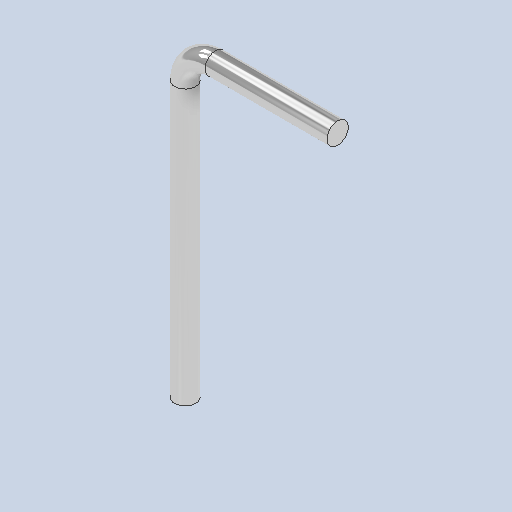
# Autodesk Inventor part: TorsOsc-202511-pin
Saved by Autodesk Inventor 2026 (Build 300175050, 175E)
## iProperties
Created: 2025-12-01
Part Number: TorsOsc-202511-pin
Material: Nickel-Copper Alloy 400
Document SubType Name: Modeling
Designer: schanen
Density: 8.83 g/cm^3
Appearance: Chrome - Polished
Author: schanen
Autodesk Inventor part; units mm, degrees
ref_plane "YZ Plane" through (0, 0, 0) normal (1, 0, 0) x (0, 1, 0)
ref_plane "XZ Plane" through (0, 0, 0) normal (0, 1, 0) x (-1, 0, 0)
ref_plane "XY Plane" through (0, 0, 0) normal (0, 0, 1) x (1, 0, 0)
sketch "Sketch1" plane through (0, 0, 0) normal (0, 0, 1) x (1, 0, 0)
  line L0 (0, 0) -> (0, 9)
  line L1 (1, 10) -> (5, 10)
  arc A0 (1, 10) -> (0, 9) centre (1, 9) ccw
  point P0 (0, 10)
  dimension "d0" = 5
  dimension "d1" = 10
  dimension "d2" = 1
  constraints: 4 end point, 2 point on circle, 2 point on line, 2 tangent, 1 centre point, 1 perpendicular, 1 vertical
  measures "d0" distance of point (0, 10) L1.end
  measures "d1" distance of L0.start point (0, 10)
  measures "d2" radius of A0
sketch "Sketch2" plane through (0, 0, 0) normal (0, 1, 0) x (-1, 0, 0)
  circle A0 centre (0, 0) radius 0.35
  dimension "d3" = 0.7
  constraints: 1 centre point, 1 coincident
  measures "d3" diameter of A0
sweep "Sweep1" add profiles "Sketch2" path "Sketch1"
body "Solid1"
